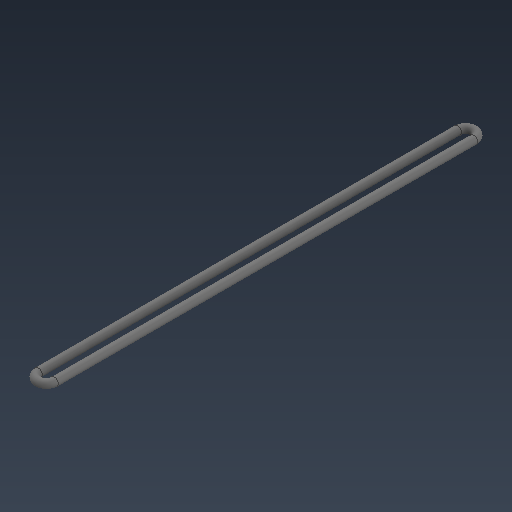
# Autodesk Inventor part: жгут сосало
Saved by Autodesk Inventor 2026 (Build 300175000, 175)
## iProperties
Created: 2026-01-20
Part Number: жгут сосало
Material: Типовые
Document SubType Name: Modeling
Designer: GameHD
Density: 1 g/cm^3
Appearance: По умолчанию
Author: GameHD
Autodesk Inventor part; units mm, degrees
ref_plane "YZ Plane" through (0, 0, 0) normal (1, 0, 0) x (0, 1, 0)
ref_plane "XZ Plane" through (0, 0, 0) normal (0, 1, 0) x (-1, 0, 0)
ref_plane "XY Plane" through (0, 0, 0) normal (0, 0, 1) x (1, 0, 0)
sketch "Эскиз1" plane through (0, 0, 0) normal (0, 0, 1) x (1, 0, 0)
  circle A0 centre (0, 0) radius 2.5
  dimension "d0" = 5
  constraints: 1 centre point, 1 coincident
  measures "d0" diameter of A0
sketch "Эскиз2" plane through (0, 0, 0) normal (0, 1, 0) x (-1, 0, 0)
  line L0 (0, 0) -> (-10, 0)
  line L1 (-5, 0) -> (-5, -260)
  line L2 (-5, 0) -> (255, 0) construction
  line L3 (-5, 0) -> (-5, -260) construction
  line L4 (-10, 0) -> (-10, -260)
  line L5 (0, -260) -> (0, 0)
  arc A0 (0, 0) -> (-10, 0) centre (-5, 0) ccw
  arc A1 (-10, -260) -> (0, -260) centre (-5, -260) ccw
  point P0 (-5, -130)
  dimension "d1" = 10
  dimension "d2" = 260
  dimension "d3" = 90
  constraints: 14 end point, 4 point on circle, 4 tangent, 3 midpoint, 2 centre point, 2 equal length, 2 horizontal, 1 perpendicular, 1 vertical
  measures "d1" distance of L0.start L0.end
  measures "d2" distance of L1.start L1.end
  measures "d3" angle of L1 L2
sweep "Сдвиг1" add profiles "Эскиз1" path "Эскиз2" path curves L5 A1 L4 A0
